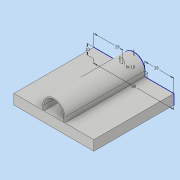
# Autodesk Inventor part: lw_5_корпус_new
Saved by Autodesk Inventor 2019 (Build 230136000, 136)
## iProperties
Created: 2021-04-29
Part Number: lw_5_корпус_new
Material: Типовые
Document SubType Name: Modeling
Designer: Kurbatova
Density: 1 g/cm^3
Appearance: По умолчанию
Author: Kurbatova
Autodesk Inventor part; units mm, degrees
ref_plane "YZ Plane" through (0, 0, 0) normal (1, 0, 0) x (0, 1, 0)
ref_plane "XZ Plane" through (0, 0, 0) normal (0, 1, 0) x (-1, 0, 0)
ref_plane "XY Plane" through (0, 0, 0) normal (0, 0, 1) x (1, 0, 0)
sketch "Эскиз9" plane through (0, 0, 0) normal (0, 0, 1) x (1, 0, 0)
  line L0 (-15, -5) -> (-5, -5)
  line L1 (0, -5) -> (-5, -5)
  line L2 (5, -5) -> (0, -5)
  line L3 (5, -5) -> (15, -5)
  line L4 (-15, -10) -> (15, -10)
  line L5 (-15, -5) -> (-15, -10)
  line L6 (-15, -5) -> (15, -5)
  line L7 (15, -10) -> (15, -5)
  line L8 (15, -10) -> (-15, -10)
  line L9 (-15, -5) -> (-15, -10)
  constraints: 20 end point, 3 collinear, 1 perpendicular
extrude "Выдавливание9" [suppressed]
sketch "Эскиз8" plane through (0, 0, 0) normal (0, 0, 1) x (1, 0, 0)
  line L0 (0, 11) -> (0, -5)
  line L1 (-11, 0) -> (11, 0)
  arc A0 (11, 0) -> (-11, 0) centre (0, 0) ccw
  line L2 (-11, 0) -> (-11, -5)
  line L3 (11, 0) -> (11, -5)
  line L4 (-10, -5) -> (-10, 0)
  arc A1 (10, 0) -> (-10, 0) centre (0, 0) ccw
  line L5 (10, 0) -> (10, -5)
  line L6 (-11, -5) -> (-10, -5)
  line L7 (10, -5) -> (11, -5)
  line L8 (11, -5) -> (40, -5)
  line L9 (-40, -5) -> (-11, -5)
  line L10 (0, -5) -> (10, -5)
  line L11 (0, -5) -> (-10, -5)
  line L12 (40, -15) -> (-40, -15)
  line L13 (-40, -15) -> (-40, -5)
  line L14 (40, -5) -> (40, -15)
  dimension "d33" = 5
  dimension "d34" = 5
  dimension "d52" = 1
  dimension "d66" = 10
  dimension "d70" = 29
  dimension "d71" = 29
  dimension "d72" = 80
  dimension "d73" = 10
  constraints: 30 end point, 6 horizontal, 5 point on circle, 3 vertical, 2 centre point, 2 tangent, 1 coincident, 1 collinear, 1 midpoint, 1 perpendicular, 1 point on line, 2 other
  measures "d33" distance of L1.start L2.end
  measures "d34" distance of L1.end L3.end
  measures "d52" radial gap between concentric circles of A0 A1
  measures "d66" radius of A1
  measures "d70" distance of L3.end L8.end
  measures "d71" distance of L9.start L2.end
  measures "d72" distance of L12.start L12.end
  measures "d73" distance of L9.start L12.end
extrude "Выдавливание17" add sketch "Эскиз8" along normal blind 80
sketch "Эскиз11" plane through (-11, -5, 0) normal (-1, 0, 0) x (0, 0, 1)
  line L0 (0, 0) -> (80, 0) projected
  line L1 (0, 5) -> (80, 5) projected
  line L2 (13.9957, 16) -> (13.9957, 0)
  line L3 (0, 0) -> (80, 0) projected
  line L4 (13.9957, 16) -> (43.9957, 16)
  line L5 (43.9957, 16) -> (43.9957, 0)
  line L6 (38.9957, 0) -> (38.9957, 9.3402)
  line L7 (38.9957, 9.3402) -> (18.9957, 9.3402)
  line L8 (18.9957, 9.3402) -> (18.9957, 0)
  line L9 (0, 5) -> (0, 5) projected
  line L10 (0, 5) -> (80, 5) projected
  line L11 (80, 5) -> (80, 5) projected
  line L12 (0, 5) -> (80, 5) projected
  dimension "d77" = 5
  dimension "d78" = 5
  dimension "d79" = 20
  constraints: 12 end point, 5 perpendicular, 4 point on line
  measures "d77" distance between parallel lines of L8 L2
  measures "d78" distance between parallel lines of L5 L6
  measures "d79" distance between parallel lines of L6 L8
extrude "Выдавливание18" cut sketch "Эскиз11" against normal blind 3 contours L2 L1 L8 L0 | L2 L4 L5 L1 L6 L7 L8 | L6 L1 L5 L0
extrude "Выдавливание19" cut sketch "Эскиз8" along normal blind 80 contours A1 L1 L0 | L0 L1 A1 | L1 L5 L10 L0 | L0 L11 L4 L1
equation "\"d66\" = diametr_"
equation "\"d77\" = diametr_ruchka_"
equation "\"d78\" = diametr_ruchka_"
equation "\"diametr_\" = 10"
equation "\"diametr_ruchka_\" = 5"
